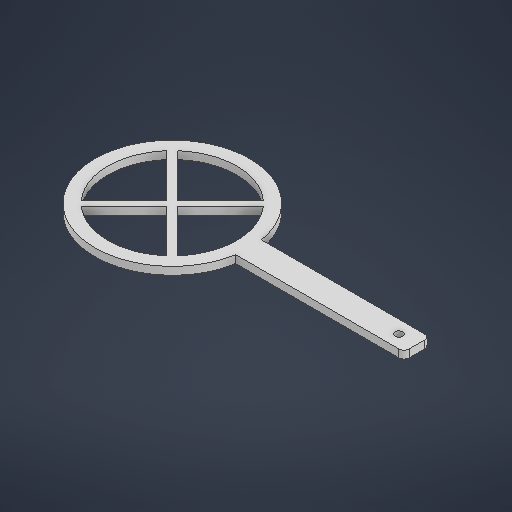
# Autodesk Inventor part: Brazo_Servo
Saved by Autodesk Inventor 2026 (Build 300175000, 175)
## iProperties
Created: 2025-06-18
Part Number: Brazo_Servo
Material: Genérico
Document SubType Name: Modeling
Designer: oscar
Density: 1 g/cm^3
Appearance: Valor por defecto
Author: oscar
Autodesk Inventor part; units mm, degrees
ref_plane "YZ Plane" through (0, 0, 0) normal (1, 0, 0) x (0, 1, 0)
ref_plane "XZ Plane" through (0, 0, 0) normal (0, 1, 0) x (-1, 0, 0)
ref_plane "XY Plane" through (0, 0, 0) normal (0, 0, 1) x (1, 0, 0)
sketch "Boceto1" plane through (0, 0, 0) normal (0, 1, 0) x (-1, 0, 0)
  line L0 (47.5, 5) -> (-47.5, 5)
  line L1 (-47.5, 5) -> (-47.5, -5)
  line L2 (-47.5, -5) -> (47.5, -5)
  line L3 (47.5, -5) -> (47.5, 5)
  line L4 (47.5, 5) -> (-47.5, -5) construction
  line L5 (-47.5, 5) -> (47.5, -5) construction
  point P0 (0, 0)
  dimension "d0" = 95
  dimension "d1" = 10
  constraints: 12 end point, 2 midpoint, 2 parallel, 1 horizontal, 1 perpendicular
  measures "d0" distance of L2.end L1.end
  measures "d1" distance of L1.end L0.end
extrude "Extrusión1" add sketch "Boceto1" along normal blind 3
sketch "Boceto2" plane through (0, 3, 0) normal (0, 1, 0) x (1, 0, 0)
  circle A0 centre (40.5, 0) radius 1.5
  line L0 (47.5, 5) -> (-47.5, 5) projected
  line L1 (47.5, -5) -> (47.5, 5) projected
  point P0 (0, 0)
  point P1 (47.5, 0)
  point P2 (47.5, 0)
  dimension "d4" = 3
  dimension "d5" = 5
  dimension "d7" = 7
  constraints: 2 midpoint, 1 centre point
  measures "d4" diameter of A0
  measures "d5" distance from line of L0 A0.centre
  measures "d7" distance of point (47.5, 0) A0.centre
extrude "Extrusión2" cut sketch "Boceto2" against normal blind 3
fillet "Empalme1" radius 2 1 edges at (-47.5, 1.5, 5)
fillet "Empalme2" radius 2 1 edges at (-47.5, 1.5, -5)
fillet "Empalme3" radius 2 1 edges at (47.5, 1.5, 5)
fillet "Empalme4" radius 2 1 edges at (47.5, 1.5, -5)
sketch "Boceto3" plane through (0, 3, 0) normal (0, 1, 0) x (1, 0, 0)
  line L0 (-47.5, 3) -> (-47.5, -3) projected
  circle A0 centre (-47.5, 0) radius 30
  line L1 (-47.5, 0) -> (-17.5, 0) construction
  line L2 (-47.5, 0) -> (-17.5, 0) construction
  point P0 (0, 0)
  dimension "d14" = 60
  constraints: 4 end point, 2 horizontal, 1 centre point, 1 midpoint
  measures "d14" diameter of A0
extrude "Extrusión3" add sketch "Boceto3" against normal blind 3
sketch "Boceto4" plane through (0, 3, 0) normal (0, 1, 0) x (1, 0, 0)
  arc A0 (-17.9196, 5) -> (-17.9196, -5) centre (-47.5, 0) ccw projected
  line L0 (-68.7649, 21.0578) -> (-8.8386, 21.0578) construction
  line L1 (-47.5, 0) -> (-26.4422, 21.0578)
  line L2 (-47.5, 0) -> (-17.7197, 0) construction
  line L3 (-47.5, 0) -> (-17.7197, 0) construction
  line L4 (-47.5, 0) -> (-68.7132, -21.2132)
  line L5 (-69.7473, 20.126) -> (-9.853, 20.126) construction
  line L6 (-59.6555, 10.0342) -> (-39.9443, -9.677)
  line L7 (-54.1333, 8.7547) -> (-36.886, -8.4927)
  line L8 (-59.6555, 10.0342) -> (-69.7473, 20.126)
  line L9 (-54.1333, 8.7547) -> (-67.626, 22.2473)
  line L10 (-36.886, -8.4927) -> (-25.2527, -20.126)
  line L11 (-39.9443, -9.677) -> (-27.374, -22.2473)
  line L12 (-69.7473, -20.126) -> (-27.374, 22.2473)
  line L13 (-25.2527, 20.126) -> (-67.626, -22.2473)
  circle A1 centre (-47.5, 0) radius 25
  point P0 (0, 0)
  point P1 (-64.0852, -18.7065)
  point P2 (-30.9148, -18.7065)
  point P3 (-47.5, -2.1213)
  point P4 (-28.7935, -16.5852)
  point P5 (-28.7935, 16.5852)
  point P6 (-45.3787, 0)
  point P7 (-30.9148, 18.7065)
  point P8 (-64.0852, 18.7065)
  point P9 (-47.5, 2.1213)
  point P10 (-66.2065, 16.5852)
  point P11 (-66.2065, -16.5852)
  point P12 (-49.6213, 0)
  dimension "d20" = 45
  dimension "d23" = 3
  dimension "d32" = 3
  dimension "d33" = 1.5
  dimension "d34" = 50
  constraints: 28 end point, 4 horizontal, 3 point on line, 2 parallel, 1 centre point, 1 coincident, 1 equal length, 10 other
  measures "d20" angle of L2 L1
  measures "d23" distance between parallel lines of L7 L6
  measures "d32" distance between parallel lines of L13 L12
  measures "d33" distance between parallel lines of L1 L12
  measures "d34" diameter of A1
extrude "Extrusión4" cut sketch "Boceto4" against normal blind 3 contours A1 L10 L7 L13 | L12 L7 L9 A1 | L6 L11 A1 L13 | L8 L6 L12 A1
